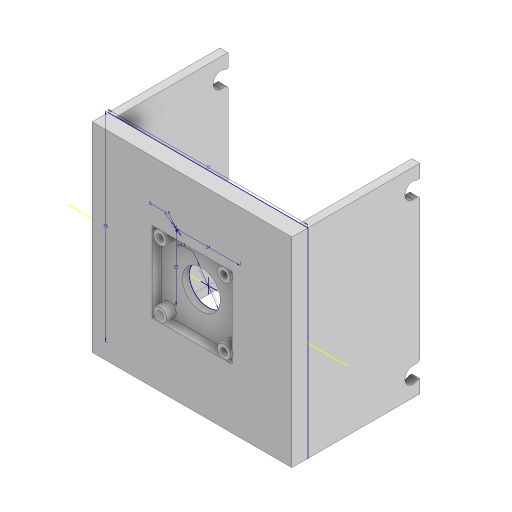
# Autodesk Inventor part: W(75mm)-camera(HBVCAM-3M2111 V22)
Saved by Autodesk Inventor 2023 (Build 270158000, 158)
## iProperties
Created: 2024-02-19
Part Number: W(75mm)-camera(HBVCAM-3M2111 V22)
Material: Generic
Document SubType Name: Modeling
Designer: N.Vladimirov
Density: 1 g/cm^3
Appearance: Default
Author: N.Vladimirov
Autodesk Inventor part; units mm, degrees
ref_plane "YZ Plane" through (0, 0, 0) normal (1, 0, 0) x (0, 1, 0)
ref_plane "XZ Plane" through (0, 0, 0) normal (0, 1, 0) x (-1, 0, 0)
ref_plane "XY Plane" through (0, 0, 0) normal (0, 0, 1) x (1, 0, 0)
sketch "Sketch1" plane through (0, 0, 0) normal (0, 0, 1) x (1, 0, 0)
  line L0 (37.5, -37.5) -> (-37.5, -37.5)
  line L1 (-37.5, -37.5) -> (-37.5, 37.5)
  line L2 (-37.5, 37.5) -> (37.5, 37.5)
  line L3 (37.5, 37.5) -> (37.5, -37.5)
  line L4 (37.5, -37.5) -> (-37.5, 37.5) construction
  line L5 (-37.5, -37.5) -> (37.5, 37.5) construction
  circle A0 centre (0, 0) radius 7.1
  circle A1 centre (-12, 12.5) radius 2.5
  circle A2 centre (-12, 12.5) radius 1.25
  line L6 (0, 2.5789) -> (0, -2.8298)
  line L7 (-2.79, 0) -> (3.5689, 0)
  circle A3 centre (12, 12.5) radius 2.5
  circle A4 centre (12, 12.5) radius 1.25
  circle A5 centre (-12, -12.5) radius 2.5
  circle A6 centre (-12, -12.5) radius 1.25
  circle A7 centre (12, -12.5) radius 2.5
  circle A8 centre (12, -12.5) radius 1.25
  line L8 (-52.5, 0) -> (52.5, 0) projected
  dimension "d0" = 75
  dimension "d1" = 75
  dimension "d2" = 14.2
  dimension "d3" = 5
  dimension "d4" = 2.5
  dimension "d7" = 24
  dimension "d10" = 25
  constraints: 16 end point, 9 centre point, 5 coincident, 2 horizontal, 2 midpoint, 2 parallel, 2 perpendicular, 2 vertical, 1 collinear, 12 other
  measures "d0" distance of L1.end L2.end
  measures "d1" distance of L0.end L1.end
  measures "d2" diameter of A0
  measures "d3" diameter of A1
  measures "d4" diameter of A2
  measures "d7" distance of A1.centre A3.centre
  measures "d10" distance of A1.centre A5.centre
extrude "Extrusion1" add sketch "Sketch1" along normal blind 2.5 contours L0 L1 L8 A0 L3 | L8 A0 L1 L2 L3
extrude "Extrusion2" add sketch "Sketch1" along normal blind 6 contours A1 | A3 | A5 | A7
sketch "Sketch2" plane through (37.5, -37.5, 0) normal (1, 0, 0) x (0, 0, -1)
  line L0 (0, -0.0252) -> (0, 75)
  arc A0 (41.0737, 69.9985) -> (39.4131, 64.5) centre (39.4131, 67.5) ccw
  arc A1 (39.4131, 10.5) -> (41.0737, 5.0015) centre (39.4131, 7.5) ccw
  line L1 (13.8443, 37.5) -> (29.6757, 37.5)
  line L2 (0, 75) -> (42, 75)
  line L3 (42, 0) -> (0, 0)
  line L4 (0, 0) -> (0, 75)
  line L5 (39.4131, 64.5) -> (41, 64.5)
  line L6 (39.4131, 10.5) -> (41, 10.5)
  line L7 (41.0737, 5.0015) -> (42, 5.0015)
  line L8 (41.0737, 69.9985) -> (42, 69.9985)
  line L9 (42, 75) -> (42, 69.9985)
  line L10 (42, 63.5) -> (42, 11.5)
  line L11 (42, 5.0015) -> (42, 0)
  arc A2 (42, 63.5) -> (41, 64.5) centre (41, 63.5) ccw
  arc A3 (41, 10.5) -> (42, 11.5) centre (41, 11.5) ccw
  point P0 (0, 37.5)
  dimension "d18" = 6
  dimension "d19" = 6
  dimension "d20" = 60
  dimension "d21" = 42
  dimension "d22" = 1
  constraints: 24 end point, 15 perpendicular, 8 point on circle, 6 tangent, 4 centre point, 4 parallel, 2 horizontal, 1 equal radius, 1 symmetric about line
  measures "d18" diameter of A0
  measures "d19" diameter of A1
  measures "d20" distance of A1.centre A0.centre
  measures "d21" distance of L3.start L3.end
  measures "d22" radius of A2
extrude "Extrusion3" add sketch "Sketch2" against normal blind 3
sketch "Sketch3" plane through (-37.5, -37.5, 0) normal (-1, 0, 0) x (0, 0, 1)
  line L0 (-41.0737, 5.0015) -> (-42, 5.0015) projected
  line L1 (-42, 5.0015) -> (-42, 0) projected
  line L2 (-42, 0) -> (0, 0) projected
  line L3 (0, 75) -> (0, 0) projected
  line L4 (0, 75) -> (-42, 75) projected
  line L5 (-42, 75) -> (-42, 69.9985) projected
  line L6 (-42, 69.9985) -> (-41.0737, 69.9985) projected
  arc A0 (-39.4131, 64.5) -> (-41.0737, 69.9985) centre (-39.4131, 67.5) ccw projected
  line L7 (-39.4131, 64.5) -> (-41, 64.5) projected
  arc A1 (-41, 64.5) -> (-42, 63.5) centre (-41, 63.5) ccw projected
  line L8 (-42, 63.5) -> (-42, 11.5) projected
  arc A2 (-42, 11.5) -> (-41, 10.5) centre (-41, 11.5) ccw projected
  line L9 (-41, 10.5) -> (-39.4131, 10.5) projected
  arc A3 (-41.0737, 5.0015) -> (-39.4131, 10.5) centre (-39.4131, 7.5) ccw projected
  point P0 (0, 37.5)
extrude "Extrusion4" add sketch "Sketch3" against normal blind 3
sketch "Sketch4" plane through (0, 0, 2.5) normal (0, 0, 1) x (1, 0, 0)
  line L0 (15, -15) -> (-15, -15)
  line L1 (-15, -15) -> (-15, 15)
  line L2 (-15, 15) -> (15, 15)
  line L3 (15, 15) -> (15, -15)
  line L4 (15, -15) -> (-15, 15) construction
  line L5 (-15, -15) -> (15, 15) construction
  line L6 (37.5, 37.5) -> (-37.5, 37.5) projected
  line L7 (-37.5, 37.5) -> (37.5, 37.5)
  line L8 (37.5, 37.5) -> (37.5, -37.5)
  line L9 (37.5, -37.5) -> (-37.5, -37.5)
  line L10 (-37.5, -37.5) -> (-37.5, 37.5)
  point P0 (0, 0)
  dimension "d27" = 30
  dimension "d28" = 30
  constraints: 20 end point, 4 parallel, 2 horizontal, 2 midpoint, 2 perpendicular
  measures "d27" distance of L1.end L2.end
  measures "d28" distance of L0.end L1.end
extrude "Extrusion5" add sketch "Sketch4" along normal up to surface (3.5 mm away)
body "Solid1"
